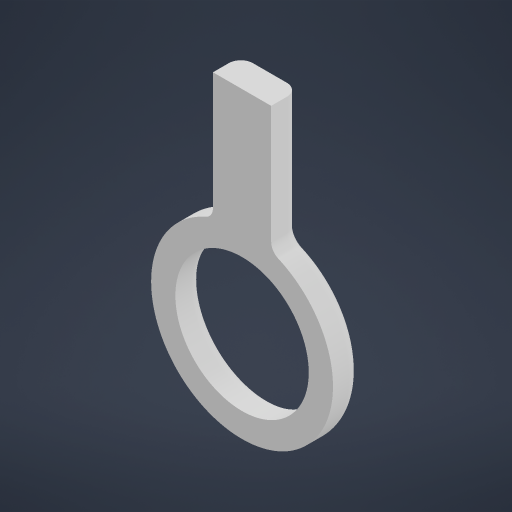
# Autodesk Inventor part: A1 Holder
Saved by Autodesk Inventor 2024.1 (Build 281209000, 209)
## iProperties
Created: 2023-09-11
Part Number: A1 Holder
Material: Generic
Document SubType Name: Modeling
Designer: User
Density: 1 g/cm^3
Appearance: Default
Author: User
Autodesk Inventor part; units mm, degrees
ref_plane "YZ Plane" through (0, 0, 0) normal (1, 0, 0) x (0, 1, 0)
ref_plane "XZ Plane" through (0, 0, 0) normal (0, 1, 0) x (-1, 0, 0)
ref_plane "XY Plane" through (0, 0, 0) normal (0, 0, 1) x (1, 0, 0)
sketch "Sketch10" plane through (0, 0, 0) normal (0, 0, 1) x (1, 0, 0)
  circle A0 centre (0, 0) radius 11
  circle A1 centre (0, 0) radius 15
  line L0 (0, 11) -> (0, 35)
  line L1 (0, 35) -> (4.8, 35)
  line L2 (4.8, 35) -> (4.8, 11)
  line L3 (4.8, 11) -> (0, 11)
  line L4 (0, 11) -> (24, 11) construction
  line L5 (4.8, 11) -> (4.8, 35)
  line L6 (4.8, 35) -> (-4.8, 35)
  line L7 (-4.8, 35) -> (-4.8, 11)
  line L8 (-4.8, 11) -> (4.8, 11)
  point P0 (-4.8, 14.2113)
  point P1 (4.8, 14.2113)
  dimension "d75" = 22
  dimension "d76" = 30
  dimension "d77" = 24
  dimension "d78" = 90
  dimension "d79" = 4.8
  dimension "d80" = 9.6
  constraints: 18 end point, 4 parallel, 4 perpendicular, 2 coincident, 1 centre point, 1 horizontal, 1 vertical, 1 vertical alignment, 2 other
  measures "d76" diameter of A1
  measures "d77" distance of L0.start L0.end
  measures "d78" angle of L4 L0
  measures "d79" distance of L0.end L1.end
  measures "d80" distance of L6.end L1.end
extrude "Extrusion8" add sketch "Sketch10" along normal blind 4.6
fillet "Fillet6" radius 2 5 edges at (4.8, 24.6056, 0) (-4.8, 24.6056, 0) (0, -15, 0) (4.8, 14.2113, 2.3) (-4.8, 14.2113, 2.3)
fillet "Fillet7" radius 2 1 edges at (-11, 0, 0)
body "Solid3"
